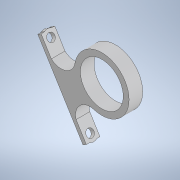
# Autodesk Inventor part: SoportePolea
Saved by Autodesk Inventor 2021 (Build 250183000, 183)
## iProperties
Created: 2022-10-28
Part Number: SoportePolea
Material: Generic
Document SubType Name: Modeling
Designer: zulet
Density: 1 g/cm^3
Appearance: Default
Mass: 3.29866 g
Surface Area: 26.1546 cm^2
Volume: 3.29866 cm^3
Author: zulet
Autodesk Inventor part; units mm, degrees
ref_plane "YZ Plane" through (0, 0, 0) normal (1, 0, 0) x (0, 1, 0)
ref_plane "XZ Plane" through (0, 0, 0) normal (0, 1, 0) x (-1, 0, 0)
ref_plane "XY Plane" through (0, 0, 0) normal (0, 0, 1) x (1, 0, 0)
sketch "Sketch1" plane through (0, 0, 0) normal (0, 0, 1) x (1, 0, 0)
  circle A0 centre (0, 0) radius 4
  circle A1 centre (0, 0) radius 11
  arc A2 (-4.0518, -13.4009) -> (-13.7956, 2.3837) centre (0, 0) ccw
  line L0 (-25.9378, -1.7681) -> (-27.6396, -2.8187) projected
  line L1 (-27.6396, -2.8187) -> (-14.9069, -23.4452) projected
  line L2 (-14.9069, -23.4452) -> (-13.205, -22.3947) projected
  arc A3 (-25.9378, -1.7681) -> (-13.7956, 2.3837) centre (-21.0023, 3.6289) ccw
  line L3 (0, 0) -> (11.913, 7.3539) construction
  arc A4 (-4.0518, -13.4009) -> (-13.205, -22.3947) centre (-6.1684, -20.4014) ccw
  dimension "d0" = 8
  dimension "d1" = 22
  dimension "d2" = 3
  dimension "d3" = 2
  constraints: 7 point on circle, 5 centre point, 2 coincident, 2 end point, 2 symmetric about line, 1 perpendicular, 1 tangent, 1 other
  measures "d0" diameter of A0
  measures "d1" diameter of A1
  measures "d2" radial gap between concentric circles of A1 A2
  measures "d3" distance from line of L0 A3.centre
extrude "Extrusion1" add sketch "Sketch1" along normal blind 7 contours A4 L2 L1 L0 A3 A2
sketch "Sketch2" plane through (-27.6396, -2.8187, 7) normal (-0.525278, 0.8509307, 0) x (0.8509307, 0.525278, 0)
  line L0 (2, 7) -> (0, 7) projected
  line L1 (0, 7) -> (0, 0) projected
  line L2 (2, 0) -> (0, 0) projected
  line L3 (2, 7) -> (2, 0) projected
  point P0 (25, 7)
extrude "Extrusion2" add sketch "Sketch2" along normal blind 10
sketch "Sketch3" plane through (-13.205, -22.3947, 0) normal (0.525278, -0.8509307, 0) x (0.8509307, 0.525278, 0)
  line L0 (-2, 0) -> (0, 0) projected
  line L1 (0, 0) -> (0, 7) projected
  line L2 (-2, 7) -> (0, 7) projected
  line L3 (-2, 0) -> (-2, 7) projected
  point P0 (23, 0)
extrude "Extrusion3" add sketch "Sketch3" along normal blind 10
sketch "Sketch4" plane through (-13.205, -22.3947, 7) normal (0.8509307, 0.525278, 0) x (0, 0, -1)
  circle A0 centre (3.5, -7) radius 2
  circle A1 centre (3.5, 31.24) radius 2
  line L0 (0, 34.24) -> (7, 34.24) projected
  line L1 (7, -10) -> (0, -10) projected
  line L2 (3.5, 31.24) -> (3.5, -7) construction
  line L3 (7, 34.24) -> (0, 34.24) projected
  line L4 (3.5, 31.24) -> (3.5, 34.24) construction
  circle A2 centre (3.5, -7) radius 3.5
  line L5 (7, 34.24) -> (7, -10) projected
  circle A3 centre (3.5, 31.24) radius 3.5
  point P0 (7, 12.12)
  point P1 (5.3028, 34.24)
  point P2 (1.6972, 34.24)
  point P3 (1.6972, -10)
  point P4 (5.3028, -10)
  dimension "d10" = 4
  dimension "d11" = 4
  dimension "d12" = 3
  dimension "d13" = 3
  constraints: 4 centre point, 4 end point, 2 coincident, 2 tangent, 2 vertical, 1 midpoint
  measures "d10" diameter of A0
  measures "d11" diameter of A1
  measures "d12" distance from line of L2.start L0
  measures "d13" distance from line of L1 L2.end
extrude "Extrusion4" cut sketch "Sketch4" against normal through all contours A0 | A1
extrude "Extrusion5" add sketch "Sketch4" against normal up to surface (2 mm away) contours A3 L0 | A2 L1 picked at (3.374, 34.3998) picked at (3.1278, -10.1057)
fillet "Fillet1" radius 2 4 edges at (-32.0415, 6.2159, 5.3028) (-32.0415, 6.2159, 1.6972) (-8.8032, -31.4293, 5.3028) (-8.8032, -31.4293, 1.6972)
equation "\"d0\" = DIR"
equation "\"d1\" = DER"
equation "\"d2\" = TB"
equation "\"d13\" = d12"
equation "\"DER\" = 22"
equation "\"HR\" = 7"
equation "\"DIR\" = 8"
equation "\"DEM\" = 4"
equation "\"Dmarc\" = 17.5"
equation "\"Bsm\" = 22.5"
equation "\"Hsm\" = 12"
equation "\"Lsm\" = 21"
equation "\"Dsc\" = 5"
equation "\"RC\" = 4"
equation "\"PB\" = 25"
equation "\"TB\" = 3"
equation "\"HSE\" = 25"
equation "\"LMaSP\" = 46.5"
body "Solid1"
